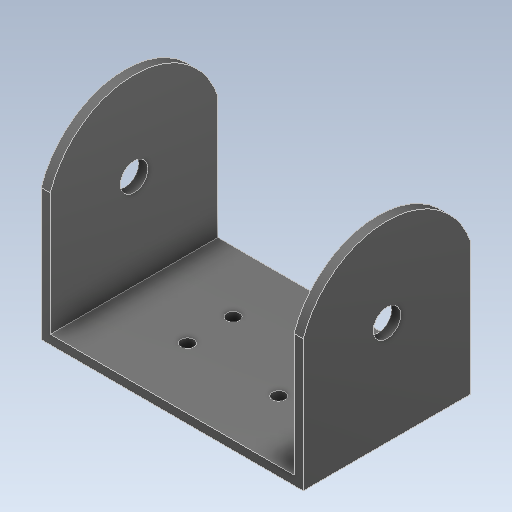
# Autodesk Inventor part: baseatas2
Saved by Autodesk Inventor 2025.1 (Build 291241000, 241)
## iProperties
Created: 2024-11-08
Part Number: baseatas2
Material: Aluminum 6061
Document SubType Name: Modeling
Designer: ramad
Density: 2.7 g/cm^3
Appearance: Aluminum - Flat
Author: ramad
Autodesk Inventor part; units mm, degrees
ref_plane "YZ Plane" through (0, 0, 0) normal (1, 0, 0) x (0, 1, 0)
ref_plane "XZ Plane" through (0, 0, 0) normal (0, 1, 0) x (-1, 0, 0)
ref_plane "XY Plane" through (0, 0, 0) normal (0, 0, 1) x (1, 0, 0)
sketch "Sketch1" plane through (0, 0, 0) normal (0, 1, 0) x (-1, 0, 0)
  line L0 (-40, 27.5) -> (40, 27.5)
  line L1 (40, 27.5) -> (40, -27.5)
  line L2 (40, -27.5) -> (-40, -27.5)
  line L3 (-40, -27.5) -> (-40, 27.5)
  line L4 (-40, 27.5) -> (40, -27.5) construction
  line L5 (40, 27.5) -> (-40, -27.5) construction
  line L6 (40, 27.5) -> (43, 27.5)
  line L7 (43, 27.5) -> (43, -27.5)
  line L8 (43, -27.5) -> (40, -27.5)
  line L9 (40, -27.5) -> (40, 27.5)
  line L10 (-40, 27.5) -> (-43, 27.5)
  line L11 (-43, 27.5) -> (-43, -27.5)
  line L12 (-43, -27.5) -> (-40, -27.5)
  line L13 (-40, -27.5) -> (-40, 27.5)
  point P0 (0, 0)
  point P1 (-40, -27.5)
  dimension "d0" = 80
  dimension "d1" = 55
  dimension "d2" = 3
  dimension "d3" = 3
  constraints: 28 end point, 6 parallel, 3 horizontal, 3 perpendicular, 2 midpoint, 1 point on line
  measures "d0" distance of L1.end L2.end
  measures "d1" distance of L0.end L1.end
  measures "d2" distance of L7.end L8.end
  measures "d3" distance of L12.end L11.end
extrude "Extrusion1" add sketch "Sketch1" along normal blind 3 contours L0 L1 L2 L3
extrude "Extrusion2" add sketch "Sketch1" along normal blind 63 contours L3 L12 L11 L10 | L6 L7 L8 L1
sketch "Sketch2" plane through (0, 3, 0) normal (0, 1, 0) x (1, 0, 0)
  line L0 (12.875, -7.5) -> (-12.875, -7.5)
  line L1 (-12.875, -7.5) -> (-12.875, 7.5)
  line L2 (-12.875, 7.5) -> (12.875, 7.5)
  line L3 (12.875, 7.5) -> (12.875, -7.5)
  line L4 (12.875, -7.5) -> (-12.875, 7.5) construction
  line L5 (-12.875, -7.5) -> (12.875, 7.5) construction
  line L6 (12.875, 7.5) -> (17.125, 7.5)
  circle A0 centre (15, 7.5) radius 2.125
  circle A1 centre (15, -7.5) radius 2.125
  line L7 (-12.875, -7.5) -> (-17.125, -7.5)
  circle A2 centre (-15, -7.5) radius 2.125
  circle A3 centre (-15, 7.5) radius 2.125
  point P0 (0, 0)
  dimension "d8" = 25.75
  dimension "d9" = 15
  dimension "d10" = 4.25
  dimension "d11" = 4.25
  constraints: 16 end point, 4 midpoint, 3 horizontal, 2 centre point, 2 horizontal alignment, 2 parallel, 1 perpendicular, 4 other
  measures "d8" distance of L1.end L2.end
  measures "d9" distance of L0.end L1.end
  measures "d10" distance of L2.end L6.end
  measures "d11" distance of L0.end L7.end
extrude "Extrusion3" cut sketch "Sketch2" against normal through all contours A2 L7 | L7 A2 | A3 | A0 L6 | L6 A0 | A1
sketch "Sketch3" plane through (-43, 0, -27.5) normal (-1, 0, 0) x (0, 0, 1)
  circle A0 centre (27.5, 34) radius 4.5
  line L0 (0, 0) -> (55, 0) projected
  circle A1 centre (27.5, 34) radius 29
  line L1 (0, 3) -> (0, 63) projected
  line L2 (0, 43.206) -> (0, 63)
  line L3 (0, 63) -> (27.5, 63)
  line L4 (55, 63) -> (0, 63) projected
  line L5 (27.5, 63) -> (55, 63)
  line L6 (55, 63) -> (55, 43.206)
  line L7 (55, 3) -> (55, 63) projected
  point P0 (27.5, 0)
  dimension "d14" = 9
  dimension "d15" = 34
  constraints: 8 end point, 2 centre point, 2 point on circle, 2 point on line, 1 coincident, 1 collinear, 1 midpoint
  measures "d14" diameter of A0
  measures "d15" distance from line of L0 A0.centre
extrude "Extrusion4" cut sketch "Sketch3" against normal through all contours A0
extrude "Extrusion5" cut sketch "Sketch3" against normal through all contours A1 L4 L6 | A1 L1 L3
body "Solid1"
